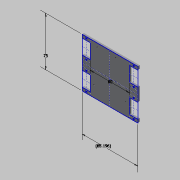
# Autodesk Inventor part: Base
Saved by Autodesk Inventor 2014 SP2 (Build 180246200, 246)
## iProperties
Created: 2015-01-06
Part Number: Base
Material: Generic
Document SubType Name: Modeling
Designer: lmarshall
Density: 1 g/cm^3
Appearance: Default
Author: lmarshall
Autodesk Inventor part; units mm, degrees
ref_plane "YZ Plane" through (0, 0, 0) normal (1, 0, 0) x (0, 1, 0)
ref_plane "XZ Plane" through (0, 0, 0) normal (0, 1, 0) x (-1, 0, 0)
ref_plane "XY Plane" through (0, 0, 0) normal (0, 0, 1) x (1, 0, 0)
sketch "Servo Hole" plane through (0, 0, 0) normal (0, 0, 1) x (1, 0, 0)
  line L0 (-67.0819, 53.6212) -> (-54.4839, 53.6212) construction
  line L1 (-54.4839, 53.6212) -> (-54.4839, 48.7062) construction
  line L2 (-54.4839, 21.2612) -> (-67.0819, 21.2612) construction
  circle A0 centre (-60.7829, 51.4432) radius 1.048
  line L3 (-67.0819, 48.7062) -> (-54.4839, 48.7062)
  line L4 (-67.0819, 26.1762) -> (-54.4839, 26.1762)
  line L5 (-54.4839, 37.4412) -> (-67.0819, 37.4412) construction
  line L6 (-54.4839, 48.7062) -> (-54.4839, 26.1762)
  line L7 (-54.4839, 26.1762) -> (-54.4839, 21.2612) construction
  line L8 (-67.0819, 48.7062) -> (-67.0819, 53.6212) construction
  line L9 (-67.0819, 26.1762) -> (-67.0819, 48.7062)
  line L10 (-67.0819, 21.2612) -> (-67.0819, 26.1762) construction
  line L11 (-60.7829, 53.6212) -> (-60.7829, 21.2612) construction
  circle A1 centre (-60.7829, 23.4392) radius 1.048
  point P0 (-60.7829, 37.4412)
  dimension "d0" = 32.36
  dimension "d2" = 2.178
  dimension "d3" = 2.096
  dimension "d4" = 22.53
  dimension "d5" = 2.096
  dimension "d6" = 2.178
  measures "d0" distance between parallel lines of L2 L0
  measures "d2" distance from line of A0.centre L0
  measures "d3" diameter of A0
  measures "d4" distance between parallel lines of L4 L3
  measures "d5" diameter of A1
  measures "d6" distance from line of L2 A1.centre
sketch "Sketch1" plane through (0, 0, 0) normal (0, 1, 0) x (-1, 0, 0)
  line L0 (-42.598, 37.5) -> (42.598, 37.5)
  line L1 (42.598, 37.5) -> (42.598, -37.5)
  line L2 (42.598, -37.5) -> (-42.598, -37.5)
  line L3 (-42.598, -37.5) -> (-42.598, 37.5)
  line L4 (-42.598, 0) -> (42.598, 0) construction
  line L5 (0, 37.5) -> (0, -37.5) construction
  line L6 (-42.598, 37.5) -> (-30, 37.5) construction
  line L7 (-30, 37.5) -> (-30, 32.585) construction
  line L8 (-30, 5.14) -> (-42.598, 5.14) construction
  circle A0 centre (-36.299, 35.322) radius 1.048
  line L9 (-42.598, 32.585) -> (-30, 32.585)
  line L10 (-42.598, 10.055) -> (-30, 10.055)
  line L11 (-30, 21.32) -> (-42.598, 21.32) construction
  line L12 (-30, 32.585) -> (-30, 10.055)
  line L13 (-30, 10.055) -> (-30, 5.14) construction
  line L14 (-42.598, 32.585) -> (-42.598, 37.5) construction
  line L15 (-42.598, 10.055) -> (-42.598, 32.585)
  line L16 (-42.598, 5.14) -> (-42.598, 10.055) construction
  line L17 (-36.299, 37.5) -> (-36.299, 5.14) construction
  circle A1 centre (-36.299, 7.318) radius 1.048
  line L18 (30, 37.5) -> (42.598, 37.5) construction
  line L19 (42.598, 37.5) -> (42.598, 32.585) construction
  line L20 (42.598, 5.14) -> (30, 5.14) construction
  circle A2 centre (36.299, 35.322) radius 1.048
  line L21 (30, 32.585) -> (42.598, 32.585)
  line L22 (30, 10.055) -> (42.598, 10.055)
  line L23 (42.598, 21.32) -> (30, 21.32) construction
  line L24 (42.598, 32.585) -> (42.598, 10.055)
  line L25 (42.598, 10.055) -> (42.598, 5.14) construction
  line L26 (30, 32.585) -> (30, 37.5) construction
  line L27 (30, 10.055) -> (30, 32.585)
  line L28 (30, 5.14) -> (30, 10.055) construction
  line L29 (36.299, 37.5) -> (36.299, 5.14) construction
  circle A3 centre (36.299, 7.318) radius 1.048
  line L30 (-42.598, -5.14) -> (-30, -5.14) construction
  line L31 (-30, -5.14) -> (-30, -10.055) construction
  line L32 (-30, -37.5) -> (-42.598, -37.5) construction
  circle A4 centre (-36.299, -7.318) radius 1.048
  line L33 (-42.598, -10.055) -> (-30, -10.055)
  line L34 (-42.598, -32.585) -> (-30, -32.585)
  line L35 (-30, -21.32) -> (-42.598, -21.32) construction
  line L36 (-30, -10.055) -> (-30, -32.585)
  line L37 (-30, -32.585) -> (-30, -37.5) construction
  line L38 (-42.598, -10.055) -> (-42.598, -5.14) construction
  line L39 (-42.598, -32.585) -> (-42.598, -10.055)
  line L40 (-42.598, -37.5) -> (-42.598, -32.585) construction
  line L41 (-36.299, -5.14) -> (-36.299, -37.5) construction
  circle A5 centre (-36.299, -35.322) radius 1.048
  line L42 (30, -5.14) -> (42.598, -5.14) construction
  line L43 (42.598, -5.14) -> (42.598, -10.055) construction
  line L44 (42.598, -37.5) -> (30, -37.5) construction
  circle A6 centre (36.299, -7.318) radius 1.048
  line L45 (30, -10.055) -> (42.598, -10.055)
  line L46 (30, -32.585) -> (42.598, -32.585)
  line L47 (42.598, -21.32) -> (30, -21.32) construction
  line L48 (42.598, -10.055) -> (42.598, -32.585)
  line L49 (42.598, -32.585) -> (42.598, -37.5) construction
  line L50 (30, -10.055) -> (30, -5.14) construction
  line L51 (30, -32.585) -> (30, -10.055)
  line L52 (30, -37.5) -> (30, -32.585) construction
  line L53 (36.299, -5.14) -> (36.299, -37.5) construction
  circle A7 centre (36.299, -35.322) radius 1.048
  point P0 (0, 0)
  point P1 (0, 0)
  dimension "d12" = 60
  dimension "d8" = 85.196
  dimension "d9" = 75
  constraints: 12 end point, 5 midpoint, 3 vertical, 1 coincident, 1 horizontal, 1 parallel, 1 perpendicular, 4 other
  measures "d8" distance between parallel lines of L1 L3
  measures "d9" distance between parallel lines of L0 L2
extrude "Extrusion1" add sketch "Sketch1" along normal blind 3 contours L0 L1 L21 L27 L22 L45 L51 L46 L2 L3 L34 L36 L33 L10 L12 L9
sketch "Sketch2" plane through (0, 3, 0) normal (0, 1, 0) x (1, 0, 0)
  line L0 (-42.598, 10.055) -> (-42.598, -10.055) projected
  line L1 (-42.598, -37.5) -> (42.598, -37.5) projected
  line L2 (42.598, -10.055) -> (42.598, 10.055) projected
  line L3 (42.598, 37.5) -> (-42.598, 37.5) projected
  line L4 (26.67, -34.29) -> (-26.67, -34.29)
  line L5 (-26.67, -34.29) -> (-26.67, 34.29)
  line L6 (-26.67, 34.29) -> (26.67, 34.29)
  line L7 (26.67, 34.29) -> (26.67, -34.29)
  circle A0 centre (-24.13, 20.32) radius 1.5
  circle A1 centre (-19.05, -31.75) radius 1.5
  circle A2 centre (24.13, 19.05) radius 1.5
  line L8 (0, 37.5) -> (0, -37.5) construction
  line L9 (42.598, 0) -> (-42.598, 0) construction
  circle A3 centre (8.89, -31.75) radius 1.5
  point P0 (0, 0)
  dimension "d18" = 3
  dimension "d19" = 2.54
  dimension "d20" = 13.97
  dimension "d21" = 53.34
  dimension "d22" = 68.58
  dimension "d23" = 3
  dimension "d24" = 7.62
  dimension "d25" = 2.54
  dimension "d28" = 3
  dimension "d29" = 2.54
  dimension "d30" = 15.24
  dimension "d31" = 3
  dimension "d32" = 27.94
  constraints: 12 end point, 4 centre point, 4 midpoint, 1 horizontal alignment, 1 perpendicular, 1 vertical, 2 other
  measures "d18" diameter of A0
  measures "d19" distance from line of A0.centre L5
  measures "d20" distance from line of A0.centre L6
  measures "d21" distance between parallel lines of L7 L5
  measures "d22" distance between parallel lines of L6 L4
  measures "d23" diameter of A1
  measures "d24" distance from line of A1.centre L5
  measures "d25" distance from line of L4 A1.centre
  measures "d28" diameter of A2
  measures "d29" distance from line of A2.centre L7
  measures "d30" distance from line of L6 A2.centre
  measures "d31" diameter of A3
  measures "d32" distance of A1.centre A3.centre
hole "Hole1" at (-24.13, 3, -20.32) at (24.13, 3, -19.05) at (8.89, 3, 31.75) at (-19.05, 3, 31.75) direction (0, -1, 0) diameter 2.459 end through all thread size "M3x0.5" class "6H" standard "ISO Metric profile"
body "Solid1"
